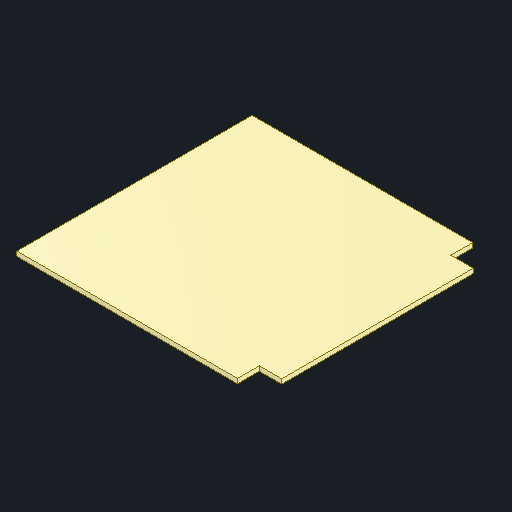
# Autodesk Inventor part: base
Saved by Autodesk Inventor 2023 (Build 270158000, 158)
## iProperties
Created: 2024-05-25
Part Number: base
Material: Nylon 6
Document SubType Name: Modeling
Designer: szymo
Density: 1.12 g/cm^3
Appearance: Nylon 6
Mass: 126.189 g
Surface Area: 669.16 cm^2
Volume: 112.668 cm^3
Author: szymo
Autodesk Inventor part; units mm, degrees
ref_plane "YZ Plane" through (0, 0, 0) normal (1, 0, 0) x (0, 1, 0)
ref_plane "XZ Plane" through (0, 0, 0) normal (0, 1, 0) x (-1, 0, 0)
ref_plane "XY Plane" through (0, 0, 0) normal (0, 0, 1) x (1, 0, 0)
sketch "Sketch1" plane through (0, 0, 0) normal (0, 1, 0) x (-1, 0, 0)
  line L0 (99, 89) -> (-99, 89)
  line L1 (-99, 89) -> (-99, -89)
  line L2 (-99, -89) -> (99, -89)
  line L3 (99, -89) -> (99, 89)
  line L4 (99, 89) -> (-99, -89) construction
  line L5 (-99, 89) -> (99, -89) construction
  line L6 (-85, 89) -> (-85, -89)
  line L7 (-68, 89) -> (-68, 72.5)
  line L8 (-68, 72.5) -> (-85, 72.5)
  line L9 (-85, -72.5) -> (-68, -72.5)
  line L10 (-68, -72.5) -> (-68, -89)
  point P0 (0, 0)
  dimension "d0" = 198
  dimension "d1" = 178
  dimension "d2" = 14
  dimension "d3" = 16.5
  dimension "d4" = 16.5
  dimension "d5" = 17
  dimension "d6" = 17
  constraints: 22 end point, 6 point on line, 4 perpendicular, 2 horizontal, 2 midpoint, 2 parallel, 1 vertical
  measures "d0" distance of L2.end L1.end
  measures "d1" distance of L1.end L0.end
  measures "d2" distance between parallel lines of L6 L1
  measures "d3" distance between parallel lines of L0 L8
  measures "d4" distance between parallel lines of L9 L2
  measures "d5" distance between parallel lines of L7 L6
  measures "d6" distance between parallel lines of L10 L6
extrude "Extrusion1" add sketch "Sketch1" along normal blind 3.5 contours L3 L2 L10 L9 L6 L8 L7 L0
body "Solid1"
